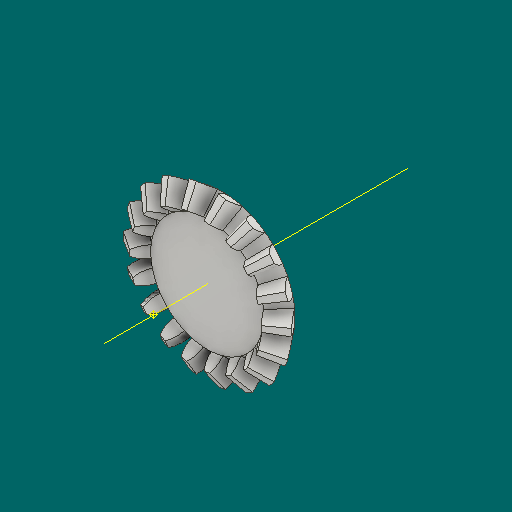
# Autodesk Inventor part: Bevel Gear1
Saved by Autodesk Inventor 2023.1 (Build 271208000, 208)
## iProperties
Created: 2022-10-10
Part Number: Bevel Gear1
Material: Steel, Mild
Document SubType Name: Modeling
Designer: zac-h
Categories: <?xml version="1.0" encoding="UTF-16"?> <MemberInstance><Categories><FamilyTemplate><FamilyTemplateParameter ValueType="xs:double" Id="1" ObjectReferenceKey="da_z" ObjectType="kUserParameterObject"/><FamilyTemplateParameter ValueType="xs:double" Id="2" ObjectReferenceKey="da_b" ObjectType="kUserParameterObject"/><FamilyTemplateParameter ValueType="xs:double" Id="3" ObjectReferenceKey="da_beta" ObjectType="kUserParameterObject"/><FamilyTemplateParameter ValueType="xs:double" Id="4" ObjectReferenceKey="da_dae" ObjectType="kUserParameterObject"/><FamilyTemplateParameter ValueType="xs:double" Id="5" ObjectReferenceKey="da_ve" ObjectType="kUserParameterObject"/><FamilyTemplateParameter ValueType="xs:double" Id="6" ObjectReferenceKey="da_omega" ObjectType="kUserParameterObject"/><FamilyTemplateParameter ValueType="xs:string" Id="7" ObjectReferenceKey="EAIAABAAAAAAHwAAAAAAAIAAAAAAAAAA" ObjectType="83914240" SubObjectId="SurfaceGeometry"/></FamilyTemplate><ParamToTemplateMap><ParamToTemplate CategoryParameter="//CategoryParameter[@InternalName='046C89C9-8512-4d59-83FE-43B91F4F132A']" TemplateParameter="1"/><ParamToTemplate CategoryParameter="//CategoryParameter[@InternalName='2552DF32-E462-4b46-AEBF-C6C7768E72AC']" TemplateParameter="2"/><ParamToTemplate CategoryParameter="//CategoryParameter[@InternalName='C9EE641D-15FC-4fae-A226-E94C4372FDD7']" TemplateParameter="3"/><ParamToTemplate><ParamToTemplate CategoryParameter="//CategoryParameter[@InternalName='00B6519A-459B-49c7-AD84-2E56D39A5744']" ConstantValue="0.000000"/></ParamToTemplate><ParamToTemplate><ParamToTemplate CategoryParameter="//CategoryParameter[@InternalName='04B31F0E-C7A6-4894-AA32-9629BEFACF47']" ConstantValue="1.000000"/></ParamToTemplate><ParamToTemplate><ParamToTemplate CategoryParameter="//CategoryParameter[@InternalName='43CBEC2E-7847-49e7-A936-2F7889FCB2D9']" ConstantValue="0.200000"/></ParamToTemplate><ParamToTemplate><ParamToTemplate CategoryParameter="//CategoryParameter[@InternalName='B1EFC894-105D-4ebd-86BF-FA20ED196853']" ConstantValue="0.266800"/></ParamToTemplate><ParamToTemplate><ParamToTemplate CategoryParameter="//CategoryParameter[@InternalName='51175063-3D10-4879-93E8-6246FE8B403D']" ConstantValue="2061532430.657340"/></ParamToTemplate><ParamToTemplate><ParamToTemplate CategoryParameter="//CategoryParameter[@InternalName='A3A52E27-4454-46a9-B0BD-C932399B70AF']" ConstantValue="0.300000"/></ParamToTemplate><ParamToTemplate CategoryParameter="//CategoryParameter[@InternalName='2A200944-5A8C-41ca-B96E-8520D2E510F1']" TemplateParameter="4"/><ParamToTemplate><ParamToTemplate CategoryParameter="//CategoryParameter[@InternalName='1A637F62-92C8-44bc-B81F-10802510B579']" ConstantValue="1.906510"/></ParamToTemplate><ParamToTemplate CategoryParameter="//CategoryParameter[@InternalName='B52DD4BE-6863-48fb-BF58-89EF6F9EC65C']" TemplateParameter="5"/><ParamToTemplate><ParamToTemplate CategoryParameter="//CategoryParameter[@InternalName='3956BFF2-84D2-457d-93C2-9B0613DEBA67']" ConstantValue="0.615807"/></ParamToTemplate><ParamToTemplate CategoryParameter="//CategoryParameter[@InternalName='739CFA02-461B-4bf8-8049-181FCAD8B28F']" TemplateParameter="6"/><ParamToTemplate><ParamToTemplate CategoryParameter="//CategoryParameter[@InternalName='A27E999F-E2CE-4481-8A2A-EBF499C4C3C5']" ConstantValue="0.000000"/></ParamToTemplate><ParamToTemplate><ParamToTemplate CategoryParameter="//CategoryParameter[@InternalName='9E1B4470-B2D3-4ff1-B813-535BB4CDF51A']" ConstantValue="3523220.976809"/></ParamToTemplate><ParamToTemplate><ParamToTemplate CategoryParameter="//CategoryParameter[@InternalName='F8452263-BFF6-458c-9FB1-07C4B99E95CD']" ConstantValue="11397033.805607"/></ParamToTemplate><ParamToTemplate><ParamToTemplate CategoryParameter="//CategoryParameter[@InternalName='3E3BB259-FD49-497f-8171-6EBC954A3479']" ConstantValue="2.000000"/></ParamToTemplate><ParamToTemplate CategoryParameter="//CategoryParameter[@InternalName='27C3BAF2-7550-4e4b-AE2C-0DB134B7D9B7']" TemplateParameter="7"/></ParamToTemplateMap><Category DisplayName="Gear" InternalName="DC85795E-93AB-48d5-8EEE-5A27447B64BD" Mnemonic="Gear"><CategoryParameter DisplayName="z" InternalName="046C89C9-8512-4d59-83FE-43B91F4F132A" Mnemonic="z"/><CategoryParameter DisplayName="b" InternalName="2552DF32-E462-4b46-AEBF-C6C7768E72AC" Mnemonic="b"/><CategoryParameter DisplayName="||b|" InternalName="C9EE641D-15FC-4fae-A226-E94C4372FDD7" Mnemonic="beta"/><CategoryParameter DisplayName="x" InternalName="00B6519A-459B-49c7-AD84-2E56D39A5744" Mnemonic="x"/><CategoryParameter DisplayName="a*" InternalName="04B31F0E-C7A6-4894-AA32-9629BEFACF47" Mnemonic="a"/><CategoryParameter DisplayName="c*" InternalName="43CBEC2E-7847-49e7-A936-2F7889FCB2D9" Mnemonic="c"/><CategoryParameter DisplayName="r|.f|*" InternalName="B1EFC894-105D-4ebd-86BF-FA20ED196853" Mnemonic="rf"/><CategoryParameter DisplayName="E" InternalName="51175063-3D10-4879-93E8-6246FE8B403D" Mnemonic="E"/><CategoryParameter DisplayName="||m|" InternalName="A3A52E27-4454-46a9-B0BD-C932399B70AF" Mnemonic="mi"/><Category DisplayName="BevelGear" InternalName="0C98F69A-0C2B-4791-B2FE-7691BB227E77" Mnemonic="BevelGear"><CategoryParameter DisplayName="d|.ae|" InternalName="2A200944-5A8C-41ca-B96E-8520D2E510F1" Mnemonic="dae"/><CategoryParameter DisplayName="d|.ai|" InternalName="1A637F62-92C8-44bc-B81F-10802510B579" Mnemonic="dai"/><CategoryParameter DisplayName="A|.e|" InternalName="B52DD4BE-6863-48fb-BF58-89EF6F9EC65C" Mnemonic="ve"/><CategoryParameter DisplayName="A|.i|" InternalName="3956BFF2-84D2-457d-93C2-9B0613DEBA67" Mnemonic="vi"/><CategoryParameter DisplayName="||S|" InternalName="739CFA02-461B-4bf8-8049-181FCAD8B28F" Mnemonic="omega"/><CategoryParameter DisplayName="x|.t|" InternalName="A27E999F-E2CE-4481-8A2A-EBF499C4C3C5" Mnemonic="xt"/><CategoryParameter DisplayName="||s||.Flim|" InternalName="9E1B4470-B2D3-4ff1-B813-535BB4CDF51A" Mnemonic="sFlim"/><CategoryParameter DisplayName="||s||.Hlim|" InternalName="F8452263-BFF6-458c-9FB1-07C4B99E95CD" Mnemonic="sHlim"/><CategoryParameter DisplayName="type" InternalName="3E3BB259-FD49-497f-8171-6EBC954A3479" Mnemonic="type"/><CategoryParameter DisplayName="PitchDiameter" InternalName="27C3BAF2-7550-4e4b-AE2C-0DB134B7D9B7" Mnemonic="IDS_PITCHDIAM"/></Category></Category></Categories></MemberInstance>
Mass: 60.9118 g
Surface Area: 34.3074 cm^2
Volume: 7.7496 cm^3
Density: 7.86 g/cm^3
Appearance: Steel
CustomPartVersion: 1
Author: zac-h
Autodesk Inventor part; units mm, degrees
ref_plane "Mesh Plane2" through (0, 0, 0) normal (0.9848078, 0.1736482, 0) x (0, 0, 1)
sketch "Teeth Body Sketch" plane through (0, 0, 0) normal (1, 0, 0) x (0, 1, 0)
  line L0 (0, 0) -> (10.4944, -10.093) construction
  line L1 (10.4944, -10.093) -> (12.2097, -7.8875)
  line L2 (12.2097, -7.8875) -> (0, 0) construction
  line L3 (11.43, -8.89) -> (0, 0) construction
  line L4 (8.1933, -7.8799) -> (9.5325, -6.1581)
  line L5 (10.4944, -10.093) -> (8.1933, -7.8799)
  line L6 (12.2097, -7.8875) -> (9.5325, -6.1581)
  line L7 (0, -11.952) -> (0, 1.992) projected
  line L8 (0, -8.89) -> (12.2097, -8.89) construction
  dimension "d0" = 22.86
  dimension "d1" = 20.9887
  dimension "d2" = 24.4194
  dimension "d3" = 3.175
  dimension "d4" = 7.8875
  constraints: 16 end point, 4 point on line, 3 perpendicular, 2 collinear, 1 horizontal alignment, 1 vertical alignment
  measures "d0" diameter of L3.start L7
  measures "d1" diameter of L0.end L7
  measures "d2" diameter of L1.end L7
  measures "d3" distance between parallel lines of L1 L4
  measures "d4" vertical distance of L1.end L0.start
revolve "Teeth Body" add sketch "Teeth Body Sketch" angle 360 about axis through (0, 0, 0) along (0, 0, 1)
ref_plane "Tooth Plane" through (0, 11.43, -8.89) normal (0, -0.7893522, 0.6139406) x (1, 0, 0)
sketch "Start Sketch" plane through (0, 11.43, -8.89) normal (0, -0.7893522, 0.6139406) x (1, 0, 0)
  line L0 (0, -24.3362) -> (0, 6.0174) projected
  arc A0 (-0.7277, -1.8593) -> (-2.2356, 1.9873) centre (-5.9621, -1.6925) ccw
  arc A1 (2.2356, 1.9873) -> (0.7277, -1.8593) centre (5.9621, -1.6925) ccw
  line L1 (-0.7277, -1.8593) -> (0.7277, -1.8593)
  arc A2 (2.2356, 1.9873) -> (-2.2356, 1.9873) centre (0, -18.6174) ccw
  dimension "d7" = 5.2371
  dimension "d8" = 5.9621
  dimension "d9" = 16.925
  dimension "d57" = 20.7256
  dimension "d58" = 16.7582
  constraints: 6 point on circle, 3 centre point, 3 symmetric about line, 2 end point, 1 coincident, 1 perpendicular, 1 other
  measures "d7" radius of A0
  measures "d8" horizontal distance of point (0, -18.617) A0.centre
  measures "d9" vertical distance of point (0, -18.617) A0.centre
  measures "d57" radius of A2
  measures "d58" distance from line of A2.centre L1
sketch "End Sketch" plane through (0, 8.8135, -6.855) normal (0, -0.7893522, 0.6139406) x (1, 0, 0)
  line L0 (0, -19.0066) -> (0, 4.6996) projected
  arc A0 (-0.5611, -1.4337) -> (-1.7239, 1.5324) centre (-4.5973, -1.305) ccw
  arc A1 (1.7239, 1.5324) -> (0.5611, -1.4337) centre (4.5973, -1.305) ccw
  line L1 (-0.5611, -1.4337) -> (0.5611, -1.4337)
  arc A2 (1.7239, 1.5324) -> (-1.7239, 1.5324) centre (0, -14.3557) ccw
  dimension "d12" = 4.0382
  dimension "d15" = 4.5973
  dimension "d16" = 13.0506
  dimension "d59" = 15.9813
  dimension "d60" = 12.922
  constraints: 6 point on circle, 3 centre point, 3 symmetric about line, 2 end point, 1 coincident, 1 other
  measures "d12" radius of A0
  measures "d15" horizontal distance of A0.centre point (0, -14.356)
  measures "d16" vertical distance of A0.centre point (0, -14.356)
  measures "d59" radius of A2
  measures "d60" distance from line of A2.centre L1
loft "Loft" cut profiles "Start Sketch", "End Sketch"
pattern_circular "Circular Pattern" count 18 over 360 about axis through (0, 0, 0) along (0, 0, 1) of "Loft"
ref_plane "End Plane" through (0, 8.8135, -6.855) normal (0, -0.7893522, 0.6139406) x (1, 0, 0)
sketch3d "3D Sketch Right"
ref_plane "End Plane Right" through (-1.0118, 8.7553, -6.855) normal (0.0906145, -0.7841339, 0.6139406) x (0.9933891, 0.1147961, 0)
sketch "End Sketch Right" plane through (-1.0118, 8.7553, -6.855) normal (0.0906145, -0.7841339, 0.6139406) x (0.9933891, 0.1147961, 0)
  arc A0 (-0.5611, -1.4337) -> (-1.7239, 1.5324) centre (-4.5973, -1.305) ccw
  line L0 (0, -19.926) -> (0, 5.619) projected
  arc A1 (1.7239, 1.5324) -> (0.5611, -1.4337) centre (4.5973, -1.305) ccw
  line L1 (-0.5611, -1.4337) -> (0.5611, -1.4337)
  arc A2 (1.7239, 1.5324) -> (-1.7239, 1.5324) centre (0, -14.3557) ccw
  dimension "d70" = 4.5973
  dimension "d71" = 13.0506
  dimension "d72" = 4.0382
  dimension "d73" = 12.922
  dimension "d74" = 15.9813
  constraints: 6 point on circle, 3 centre point, 3 symmetric about line, 2 end point, 1 coincident, 1 perpendicular, 1 other
  measures "d70" horizontal distance of A2.centre A0.centre
  measures "d71" vertical distance of point (0, -14.356) A0.centre
  measures "d72" radius of A0
  measures "d73" distance from line of point (0, -14.356) L1
  measures "d74" radius of A2
feature "Loft Right" [suppressed]
pattern_circular "Circular Pattern Right" [suppressed]
sketch3d "3D Sketch Left"
ref_plane "End Plane Left" through (1.0339, 8.7553, -6.8661) normal (-0.0925205, -0.7835118, 0.6144504) x (0.9931001, -0.1172697, 0)
sketch "End Sketch Left" plane through (1.0339, 8.7553, -6.8661) normal (-0.0925205, -0.7835118, 0.6144504) x (0.9931001, -0.1172697, 0)
  line L0 (0, -20.9883) -> (0, 6.6984) projected
  arc A0 (-0.5611, -1.4265) -> (-1.7239, 1.5396) centre (-4.5973, -1.2978) ccw
  arc A1 (1.7239, 1.5396) -> (0.5611, -1.4265) centre (4.5973, -1.2978) ccw
  line L1 (-0.5611, -1.4265) -> (0.5611, -1.4265)
  ellipse E0 centre (0, -4.8584) end of major axis (9.5325, -4.8584) minor radius 5.8573 projected
  arc A2 (1.7239, 1.5396) -> (-1.7239, 1.5396) centre (0, -14.3485) ccw
  dimension "d56" = 5.8573
  dimension "d30" = 4.0382
  dimension "d31" = 4.5973
  dimension "d32" = 13.0506
  dimension "d61" = 15.9813
  dimension "d62" = 12.922
  constraints: 6 point on circle, 3 centre point, 3 symmetric about line, 2 end point, 1 coincident, 2 other
  measures "d30" radius of A0
  measures "d31" horizontal distance of point (0, -14.348) A0.centre
  measures "d32" vertical distance of A0.centre point (0, -14.348)
  measures "d61" radius of A2
  measures "d62" distance from line of point (0, -14.348) L1
feature "Loft Left" [suppressed]
pattern_circular "Circular Pattern Left" [suppressed]
sketch "Body Sketch" plane through (0, 0, 0) normal (1, 0, 0) x (0, 1, 0)
  line L0 (0, -10.3816) -> (0, -7.4302) projected
  line L1 (10.4944, -10.093) -> (8.1933, -7.8799) projected
  line L2 (8.1933, -7.8799) -> (0, -7.8799)
  line L3 (10.4944, -10.093) -> (0, -10.093)
  constraints: 4 end point, 2 perpendicular, 2 point on line
revolve "Fix Body" add sketch "Body Sketch" angle 360 about axis through (0, 0, 0) along (0, 0, 1)
sketch "Sketch6" plane through (0, 0, 0) normal (1, 0, 0) x (0, 1, 0)
  line L0 (11.43, -8.89) -> (0, 0) projected
  line L1 (0, -10.8) -> (0, 1.8) projected
surface revolve "Pitch Diameter" sketch "Sketch6" angle 360 about axis through (0, 0, 0) along (0, 0, 1) shown no curves L0
equation "\"d0\" = da_de"
equation "\"d1\" = da_dfe"
equation "\"d2\" = da_dae"
equation "\"d3\" = da_b"
equation "\"d4\" = da_ve"
equation "\"d7\" = fd_rr"
equation "\"d8\" = fd_x"
equation "\"d9\" = fd_y"
equation "\"d57\" = 0.5 * fd_dva + 0.3 * da_he"
equation "\"d58\" = 0.5 * fd_dva - 1.12 * da_he"
equation "\"da_teethtype\" = 0"
equation "\"da_b\" = 3.175"
equation "\"da_de\" = 22.86"
equation "\"da_dae\" = 24.41941"
equation "\"da_dfe\" = 20.98871"
equation "\"da_le\" = 14.48023"
equation "\"da_omega\" = 90deg"
equation "\"da_beta\" = 0"
equation "\"da_delta\" = 52.125016deg"
equation "\"da_alpha\" = 14.5deg"
equation "\"da_he\" = 2.794"
equation "\"da_ve\" = 7.88752"
equation "\"da_zv\" = 29.318797"
equation "\"fd_loft\" = da_b + 0.05 * da_he"
equation "\"fd_x\" = fd_x1 + fd_x2"
equation "\"fd_y\" = fd_y1 - fd_y2"
equation "\"fd_dd\" = fd_dva - 0.8 * da_he"
equation "\"da_dvw\" = 37.23487"
equation "\"d11\" = fd_loft"
equation "\"da_dm\" = 20.35381"
equation "\"da_x\" = 0"
equation "\"da_m\" = 1.27"
equation "\"d50\" = da_omega"
equation "\"fd_rr\" = 5.237059"
equation "\"fd_dva\" = 39.774872"
equation "\"fd_x1\" = 0.996979"
equation "\"fd_x2\" = 4.965088"
equation "\"fd_y1\" = 18.590722"
equation "\"fd_y2\" = 1.665739"
body "Solid1"
body "Srf1"
